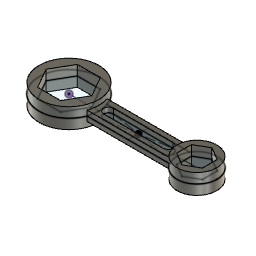
exercise2 (Autodesk Fusion 360 design; units mm, degrees)
Autodesk Fusion 360 part; units mm, degrees
sketch "Sketch2" plane through (0, 0, 0) normal (0, 0, 1) x (1, 0, 0)
  circle A0 centre (0, 0) radius 30
  circle A1 centre (129, 0) radius 20
  line L0 (28.2843, 10) -> (111.6795, 10)
  line L1 (0, 0) -> (129, 0)
  line L2 (28.2843, -10) -> (111.6795, -10)
  line L3 (-11.547, 20) -> (-23.094, 0)
  line L4 (-23.094, 0) -> (-11.547, -20)
  line L5 (-11.547, -20) -> (11.547, -20)
  line L6 (11.547, -20) -> (23.094, 0)
  line L7 (23.094, 0) -> (11.547, 20)
  line L8 (11.547, 20) -> (-11.547, 20)
  line L9 (129, 15) -> (116.0096, 7.5)
  line L10 (116.0096, 7.5) -> (116.0096, -7.5)
  line L11 (116.0096, -7.5) -> (129, -15)
  line L12 (129, -15) -> (141.9904, -7.5)
  line L13 (141.9904, -7.5) -> (141.9904, 7.5)
  line L14 (141.9904, 7.5) -> (129, 15)
  line L15 (39.9819, 5) -> (99.9819, 5)
  line L16 (99.9819, -5) -> (39.9819, -5)
  line L17 (39.9819, 5) -> (99.9819, -5) construction
  line L18 (39.9819, -5) -> (99.9819, 5) construction
  line L19 (69.9819, 10) -> (69.9819, -10) construction
  arc A2 (39.9819, 5) -> (39.9819, -5) centre (39.9819, 0) ccw
  arc A3 (99.9819, -5) -> (99.9819, 5) centre (99.9819, 0) ccw
  point P0 (129, 0)
  point P1 (69.9819, 0)
  dimension "d12" = 129
  dimension "d13" = 60
  dimension "d14" = 40
  dimension "d15" = 20
  dimension "d16" = 20
  dimension "d17" = 15
  dimension "d18" = 60
  dimension "d19" = 10
  dimension "d20" = 5
  dimension "d21" = 5
  constraint coincident A0.centre L1.start
  constraint coincident A0 L0.start
  constraint coincident A1 L0.end
  constraint horizontal L0
  constraint coincident P0 A1.centre
  constraint parallel L0 L1
  constraint coincident A0 L2.start
  constraint coincident A1 L2.end
  constraint horizontal L2
  constraint equal L0 L2
  constraint horizontal L8
  constraint vertical P0 L9.start
  constraint horizontal L15
  constraint horizontal L16
  constraint midpoint L18 P1
  constraint horizontal A0.centre P1
  constraint midpoint L0 L19.start
  constraint midpoint L2 L19.end
  constraint vertical P1 L19.start
  measures "d12" distance of A0.centre P0
  measures "d13" diameter of A0
  measures "d14" diameter of A1
  measures "d15" distance of L0 L2
  measures "d16" distance of A0.centre L8
  measures "d17" distance of L9.start P0
  measures "d18" distance of L16.start L16.end
  measures "d19" distance of L15.end L16.start
  measures "d20" radius of A2
  measures "d21" radius of A3
extrude "Extrude3" add sketch "Sketch2" along normal mid plane 20 contours A0 | A1 makes body 1 at (27.1662, -12.7278, 3.3333) makes body 2 at (148.9006, -1.9914, -3.3333)
extrude "Extrude4" add sketch "Sketch2" along normal mid plane 10 contours A0 A1 L1 L2 L16 A2 A3 | A0 A1 L0 L1 L15 A2 A3 bodies 1 2
